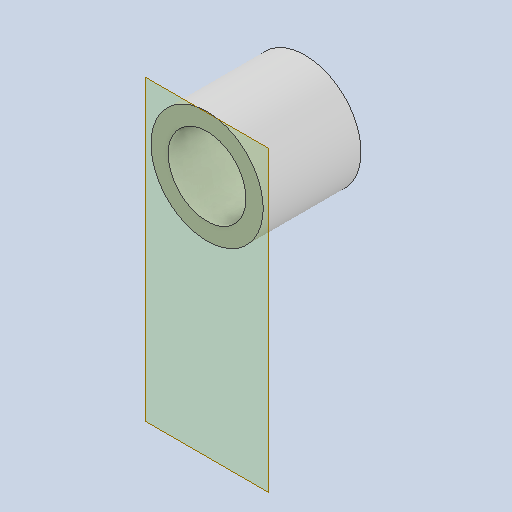
# Autodesk Inventor part: spacerB_V3
Saved by Autodesk Inventor 2023 (Build 270158000, 158)
## iProperties
Created: 2022-11-25
Part Number: spacerB_V3
Material: Generic
Document SubType Name: Modeling
Designer: shrey
Density: 1 g/cm^3
Appearance: Default
Author: shrey
Autodesk Inventor part; units mm, degrees
ref_plane "YZ Plane" through (0, 0, 0) normal (1, 0, 0) x (0, 1, 0)
ref_plane "XZ Plane" through (0, 0, 0) normal (0, 1, 0) x (-1, 0, 0)
ref_plane "XY Plane" through (0, 0, 0) normal (0, 0, 1) x (1, 0, 0)
ref_plane "Work Plane1" through (-28.7191, -12.6033, -39.9821) normal (0, 0, -1) x (-1, 0, 0)
sketch "Sketch1" plane through (-28.7191, -12.6033, -39.9821) normal (0, 0, -1) x (-1, 0, 0)
  circle A0 centre (-10.5928, 20.0161) radius 9.16 projected
  circle A1 centre (-10.5928, 20.0161) radius 6.36 projected
  point P0 (-28.7191, 12.6033)
extrude "Extrusion1" add sketch "Sketch1" along normal blind 16
body "Solid1"
